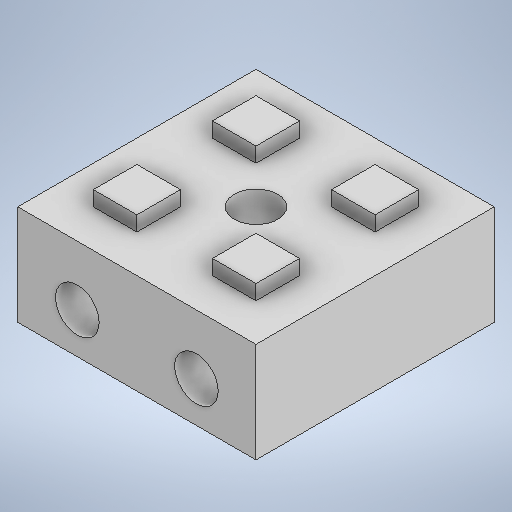
# Autodesk Inventor part: odom connector
Saved by Autodesk Inventor 2025.1 (Build 291241020, 241B)
## iProperties
Created: 2025-01-13
Part Number: odom connector
Material: Generic
Document SubType Name: Modeling
Designer: AtuStem
Density: 1 g/cm^3
Appearance: Default
Author: AtuStem
Autodesk Inventor part; units mm, degrees
ref_plane "YZ Plane" through (0, 0, 0) normal (1, 0, 0) x (0, 1, 0)
ref_plane "XZ Plane" through (0, 0, 0) normal (0, 1, 0) x (-1, 0, 0)
ref_plane "XY Plane" through (0, 0, 0) normal (0, 0, 1) x (1, 0, 0)
sketch "Sketch1" plane through (0, 0, 0) normal (0, 1, 0) x (-1, 0, 0)
  line L0 (0, 0) -> (25.4, 0)
  line L1 (25.4, 0) -> (25.4, 25.4)
  line L2 (25.4, 25.4) -> (0, 25.4)
  line L3 (0, 25.4) -> (0, 0)
  line L4 (12.7, 25.4) -> (12.7, 0)
  line L5 (12.7, 25.4) -> (38.1, 25.4) construction
  line L6 (0, 12.7) -> (25.4, 12.7)
  line L7 (0, 12.7) -> (25.4, 12.7) construction
  line L8 (12.7, 6.35) -> (25.4, 6.35)
  line L9 (12.7, 6.35) -> (25.4, 6.35) construction
  line L10 (19.05, 0) -> (19.05, 12.7)
  line L11 (16.7259, 16.7259) -> (21.3741, 16.7259)
  line L12 (21.3741, 16.7259) -> (21.3741, 21.3741)
  line L13 (21.3741, 21.3741) -> (16.7259, 21.3741)
  line L14 (16.7259, 21.3741) -> (16.7259, 16.7259)
  line L15 (16.7259, 16.7259) -> (19.05, 19.05) construction
  line L16 (21.3741, 16.7259) -> (16.7259, 21.3741) construction
  line L17 (8.6741, 16.7259) -> (8.6741, 21.3741)
  line L18 (8.6741, 21.3741) -> (4.0259, 21.3741)
  line L19 (4.0259, 21.3741) -> (4.0259, 16.7259)
  line L20 (4.0259, 16.7259) -> (8.6741, 16.7259)
  line L21 (21.3741, 4.0259) -> (21.3741, 8.6741)
  line L22 (21.3741, 8.6741) -> (16.7259, 8.6741)
  line L23 (16.7259, 8.6741) -> (16.7259, 4.0259)
  line L24 (16.7259, 4.0259) -> (21.3741, 4.0259)
  line L25 (8.6741, 4.0259) -> (8.6741, 8.6741)
  line L26 (8.6741, 8.6741) -> (4.0259, 8.6741)
  line L27 (4.0259, 8.6741) -> (4.0259, 4.0259)
  line L28 (4.0259, 4.0259) -> (8.6741, 4.0259)
  circle A0 centre (12.7, 12.7) radius 2.3241
  dimension "d0" = 25.4
  dimension "d1" = 25.4
  dimension "d2" = 25.4
  dimension "d3" = 90
  dimension "d4" = 25.4
  dimension "d5" = 0
  dimension "d6" = 12.7
  dimension "d7" = 0
  dimension "d8" = 4.6482
  dimension "d9" = 4.6482
  dimension "d12" = 12.7
  dimension "d15" = 12.7
  dimension "d18" = 4.6482
  constraints: 58 end point, 7 horizontal, 5 midpoint, 5 perpendicular, 4 parallel, 3 equal length, 2 point on line, 1 centre point, 1 vertical, 24 other
  measures "d0" distance of L2.end L1.end
  measures "d1" distance of L1.end L0.end
  measures "d2" distance of L4.start L4.end
  measures "d3" angle of L4 L5
  measures "d4" distance of L6.start L6.end
  measures "d5" distance between parallel lines of L6 L7
  measures "d6" distance of L8.start L8.end
  measures "d7" distance between parallel lines of L8 L9
  measures "d8" distance of L13.end L12.end
  measures "d9" distance of L12.end L11.end
  measures "d12" distance of L11.end L17.start
  measures "d15" distance of L11.end L21.start
  measures "d18" diameter of A0
extrude "Extrusion1" add sketch "Sketch1" along normal blind 1.5875 contours L24 L23 L8 L10 | L10 L8 L21 L24 | L23 L22 L10 L8 | L10 L22 L21 L8 | L14 L13 L12 L11 | L20 L19 L18 L17 | L28 L27 L26 L25
extrude "Extrusion2" add sketch "Sketch1" against normal blind 10.668 contours L3 L6 A0 L4 L0 | L4 L8 L23 L24 L10 L0 | L3 L2 L4 A0 L6 | L10 L24 L21 L8 L1 L0 | L4 A0 L6 L10 L22 L23 L8 | A0 L4 L6 | L6 L4 A0 | L24 L23 L8 L10 | L10 L8 L21 L24 | L4 L6 A0 | L23 L22 L10 L8 | L2 L1 L6 A0 L4 | L4 A0 L6 | L8 L21 L22 L10 L6 L1 | L10 L22 L21 L8 | L14 L13 L12 L11 | L20 L19 L18 L17 | L28 L27 L26 L25
hole "Hole1" at (-12.7, 0, 12.7) direction (0, -1, 0) diameter 4.6482 depth 32.3342 tip angle 118
sketch "Sketch2" plane through (0, 0, 0) normal (0, 0, -1) x (-1, 0, 0)
  line L0 (25.4, 0) -> (0, 0) projected
  line L1 (25.4, 0) -> (0, 0)
  line L2 (12.7, 2.032) -> (12.7, -10.668)
  line L3 (15.0241, -10.668) -> (10.3759, -10.668) projected
  line L4 (12.7, -5.334) -> (25.4, -5.334)
  line L5 (25.4, 0) -> (25.4, -10.668) projected
  line L6 (12.7, -5.334) -> (0, -5.334)
  line L7 (0, 0) -> (0, -10.668) projected
  circle A0 centre (19.05, -6.35) radius 2.3241
  circle A1 centre (6.35, -6.35) radius 2.3241
  dimension "d30" = 4.6482
  constraints: 8 end point, 3 midpoint, 2 centre point, 1 horizontal, 1 symmetric about line, 1 other
  measures "d30" diameter of A0
extrude "Extrusion3" cut sketch "Sketch2" against normal through all contours A0 L4 | L4 A0 | A1 L6 | L6 A1
body "Solid1"
